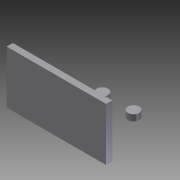
# Autodesk Inventor part: USB A block
Saved by Autodesk Inventor 2012 (Build 160160000, 160)
## iProperties
Created: 2017-04-26
Part Number: USB A block
Material: Default
Document SubType Name: Modeling
Designer: Brandon
Density: 1 g/cm^3
Author: Brandon
Autodesk Inventor part; units mm, degrees
ref_plane "YZ Plane" through (0, 0, 0) normal (1, 0, 0) x (0, 1, 0)
ref_plane "XZ Plane" through (0, 0, 0) normal (0, 1, 0) x (-1, 0, 0)
ref_plane "XY Plane" through (0, 0, 0) normal (0, 0, 1) x (1, 0, 0)
sketch "Sketch1" plane through (0, 0, 0) normal (0, 0, 1) x (1, 0, 0)
  line L0 (-8, 4.25) -> (8, 4.25)
  line L1 (8, 4.25) -> (8, -4.25)
  line L2 (8, -4.25) -> (-8, -4.25)
  line L3 (-8, -4.25) -> (-8, 4.25)
  point P0 (0, 0)
  dimension "d0" = 16
  dimension "d1" = 8.5
  dimension "d2" = 8
  dimension "d3" = 4.25
  constraints: 8 end point, 2 parallel, 1 horizontal, 1 perpendicular
  measures "d0" distance of L0.start L0.end
  measures "d1" distance of L2.end L0.start
  measures "d2" distance from line of point (0, 0) L3
  measures "d3" distance from line of L0 point (0, 0)
extrude "Extrusion1" add sketch "Sketch1" along normal blind 1
sketch "Sketch3" plane through (-8, -4.25, 0) normal (0, -1, 0) x (1, 0, 0)
  line L0 (16, 1) -> (0, 1) projected
  circle A0 centre (5.5, -8.9) radius 0.9
  circle A1 centre (10.5, -8.9) radius 0.9
  point P0 (8, 0)
  dimension "d6" = 1.8
  dimension "d7" = 1.8
  dimension "d8" = 5
  dimension "d9" = 2.5
  dimension "d10" = 9.9
  constraints: 2 centre point
  measures "d6" diameter of A0
  measures "d7" diameter of A1
  measures "d8" distance of A1.centre A0.centre
  measures "d9" horizontal distance of point (8, 0) A0.centre
  measures "d10" distance from line of L0 A0.centre
extrude "Extrusion2" add sketch "Sketch3" along normal blind 1
equation "\"d2\" = 0.5 * d0"
equation "\"d3\" = 0.5 * d1"
body "Solid1"
